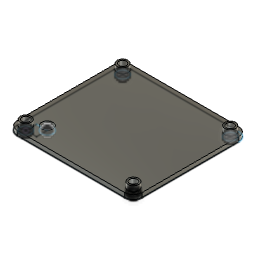
orangepi_parts (Autodesk Fusion 360 design; units mm, degrees)
Autodesk Fusion 360 part; units mm, degrees
note: some values were not read from the file. Set by a fixed rule: which sketch regions a step uses.
sketch "Sketch1" plane through (0, 0, 0) normal (0, 0, 1) x (1, 0, 0)
  circle A0 centre (0, 45) radius 1.75
  circle A1 centre (50, 45) radius 1.75
  circle A2 centre (0, 0) radius 1.75
  circle A3 centre (50, 0) radius 1.75
  line L0 (54, 45) -> (54, 0)
  line L1 (-4, 0) -> (-4, 45)
  line L2 (0, 49) -> (50, 49)
  line L3 (50, -4) -> (0, -4)
  line L4 (-1.75, 45) -> (1.75, 45)
  line L5 (48.25, 45) -> (51.75, 45)
  line L6 (50, 45) -> (48.25, 45)
  line L7 (1.75, 45) -> (0, 45)
  line L8 (0, -1.75) -> (0, 1.75)
  line L9 (0, 43.25) -> (0, 46.75)
  line L10 (0, 45) -> (0, 43.25)
  line L11 (0, 1.75) -> (0, 0)
  arc A4 (0, 49) -> (-4, 44.9977) centre (0, 45) ccw
  line L12 (50, 46.75) -> (50, 43.25)
  line L13 (50, 1.75) -> (50, -1.75)
  line L14 (50, 0) -> (50, 1.75)
  line L15 (50, 43.25) -> (50, 45)
  arc A5 (54, 45) -> (50, 49) centre (50, 45) ccw
  arc A6 (50, -4) -> (54, 0) centre (50, 0) ccw
  line L16 (0, 0) -> (1.75, 0)
  line L17 (48.25, 0) -> (50, 0)
  line L18 (51.75, 0) -> (48.25, 0)
  line L19 (1.75, 0) -> (-1.75, 0)
  arc A7 (-4, 0) -> (0, -4) centre (0, 0) ccw
  circle A8 centre (0, 0) radius 2.5
  circle A9 centre (0, 45) radius 2.5
  circle A10 centre (50, 45) radius 2.5
  circle A11 centre (50, 0) radius 2.5
  line L20 (0, 0) -> (5, 0)
  line L21 (5, 0) -> (5, 5)
  line L22 (5, 5) -> (0, 5)
  line L23 (0, 5) -> (0, 0)
  circle A12 centre (5, 5) radius 2.625
  dimension "d1" = 50
  dimension "d2" = 45
  dimension "d3" = 3.5
  dimension "d4" = 3.5
  dimension "d5" = 3.5
  dimension "d6" = 3.5
  dimension "d7" = 8
  dimension "d9" = 8
  dimension "d10" = 8
  dimension "d11" = 5
  dimension "d12" = 5
  dimension "d13" = 5
  dimension "d14" = 5
  dimension "d19" = 5
  dimension "d20" = 5.25
  constraint horizontal L16
  constraint vertical L14
  constraint horizontal L6
  constraint vertical L10
  constraint coincident A2.centre L11.end
  constraint coincident A0.centre L7.end
  constraint coincident A1.centre L6.start
  constraint coincident A3.centre L14.start
  constraint concentric A0 A4
  constraint concentric A3 A6
  constraint horizontal L4
  constraint vertical L0
  constraint horizontal L18
  constraint vertical L1
  constraint coincident L1.end A4
  constraint horizontal L2
  constraint vertical L12
  constraint horizontal L3
  constraint vertical L8
  constraint collinear L4 L5
  constraint collinear L6 L7
  constraint coincident A0 L4.end
  constraint collinear L8 L9
  constraint collinear L10 L11
  constraint coincident L1 A4.end
  constraint coincident A0 L9.start
  constraint coincident A1 L5.start
  constraint coincident A1 L12.end
  constraint collinear L12 L13
  constraint collinear L14 L15
  constraint coincident A3 L13.start
  constraint coincident A3 L17.start
  constraint collinear L16 L17
  constraint collinear L18 L19
  constraint coincident A2 L16.end
  constraint coincident A2 L8.end
  constraint coincident A0 L9.end
  constraint coincident A0 L4.start
  constraint coincident A1 L12.start
  constraint coincident A1 L5.end
  constraint coincident A3 L18.start
  constraint coincident A3 L13.end
  constraint coincident A2 L8.start
  constraint coincident A2 L19.end
  constraint concentric A6 A11
  constraint horizontal L20
  constraint vertical L21
  constraint horizontal L22
  constraint vertical L23
  constraint coincident L21.end L22.start
  measures "d1" distance of A2.centre A3.centre
  measures "d2" distance of A2.centre A0.centre
  measures "d3" diameter of A0
  measures "d4" diameter of A1
  measures "d5" diameter of A2
  measures "d6" diameter of A3
  measures "d7" diameter of A4
  measures "d9" diameter of A7
  measures "d10" diameter of A6
  measures "d11" diameter of A8
  measures "d12" diameter of A9
  measures "d13" diameter of A10
  measures "d14" diameter of A11
  measures "d19" distance of A2.centre L20.end
  measures "d20" diameter of A12
extrude "Extrude1" add sketch "Sketch1" along normal blind 2 contours A8 L20 L21 L22 L23 A12 | L21 L22 A12 | L21 L22 A12 | L0 L1 L2 L3 A4 A5 A6 A7
extrude "Extrude2" add sketch "Sketch1" along normal blind 4.5 contours A2 A8 L20 L23 | A2 A8 L20 L23 | A9 | A10 | A11
extrude "Extrude3" cut sketch "Sketch1" along normal blind 10 contours L21 L22 A12 | L21 L22 A12
